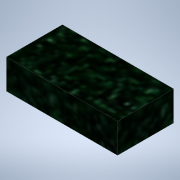
# Autodesk Inventor part: BAKUSO
Saved by Autodesk Inventor 2020.2 (Build 242310000, 310)
## iProperties
Created: 2019-03-09
Part Number: BAKUSO
Material: 一般
Document SubType Name: Modeling
Designer: mozar
Density: 1.70791 g/cm^3
Appearance: 芝生 - イチゴツナギ
Mass: 184 g
Surface Area: 156.345 cm^2
Volume: 107.734 cm^3
Author: mozar
Autodesk Inventor part; units mm, degrees
ref_plane "YZ Plane" through (0, 0, 0) normal (1, 0, 0) x (0, 1, 0)
ref_plane "XZ Plane" through (0, 0, 0) normal (0, 1, 0) x (-1, 0, 0)
ref_plane "XY Plane" through (0, 0, 0) normal (0, 0, 1) x (1, 0, 0)
sketch "スケッチ1" plane through (0, 0, 0) normal (0, 0, 1) x (1, 0, 0)
  line L0 (0, 0) -> (93, 0)
  line L1 (93, 0) -> (93, 46.9)
  line L2 (93, 46.9) -> (0, 46.9)
  line L3 (0, 46.9) -> (0, 0)
  dimension "d0" = 93
  dimension "d1" = 46.9
  constraints: 8 end point, 2 parallel, 1 horizontal, 1 perpendicular
  measures "d0" distance of L2.end L1.end
  measures "d1" distance of L1.end L0.end
extrude "押し出し1" add sketch "スケッチ1" along normal blind 24.7
sketch "スケッチ3" plane through (0, 0, 0) normal (0, 0, -1) x (-1, 0, 0)
  line L0 (0, 46.9) -> (0, 0) projected
  line L1 (0, 0) -> (-93, 0) projected
  line L2 (-93, 0) -> (-93, 46.9) projected
  line L3 (-93, 46.9) -> (0, 46.9) projected
